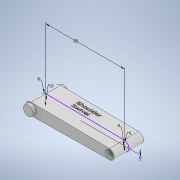
# Autodesk Inventor part: shoulder swivel
Saved by Autodesk Inventor 2020 (Build 240168000, 168)
## iProperties
Created: 2020-12-23
Part Number: shoulder swivel
Material: Generic
Document SubType Name: Modeling
Designer: frost
Density: 1 g/cm^3
Appearance: Default
Author: frost
Autodesk Inventor part; units mm, degrees
ref_plane "YZ Plane" through (0, 0, 0) normal (1, 0, 0) x (0, 1, 0)
ref_plane "XZ Plane" through (0, 0, 0) normal (0, 1, 0) x (-1, 0, 0)
ref_plane "XY Plane" through (0, 0, 0) normal (0, 0, 1) x (1, 0, 0)
sketch "Sketch1" plane through (0, 0, 0) normal (0, 0, 1) x (1, 0, 0)
  line L0 (0, 0) -> (-34.9606, 0)
  circle A0 centre (-34.9606, 0) radius 5
  circle A1 centre (45.0394, 0) radius 4
  arc A2 (-34.8856, 5.9995) -> (-34.8856, -5.9995) centre (-34.9606, 0) ccw
  arc A3 (45.1019, -4.9996) -> (45.1019, 4.9996) centre (45.0394, 0) ccw
  line L1 (-34.8856, 5.9995) -> (45.1019, 4.9996)
  line L2 (-34.8856, -5.9995) -> (45.1019, -4.9996)
  line L3 (-34.9606, 0) -> (-29.9606, 0)
  line L4 (-34.9606, 0) -> (-12.8373, 0)
  dimension "d7" = 10
  dimension "d6" = 6
  dimension "d8" = 8
  dimension "d9" = 5
  dimension "d10" = 80
  dimension "d15" = 0
  constraints: 10 end point, 4 point on circle, 4 tangent, 3 centre point, 3 coincident, 2 horizontal, 1 horizontal alignment, 1 point on line, 2 other
  measures "d6" radius of A2
  measures "d8" diameter of A1
  measures "d9" radius of A3
  measures "d10" distance of point (-34.961, 0) A1.centre
  measures "d15" distance from line of A1.centre L0
extrude "Extrusion1" add sketch "Sketch1" along normal mid plane 30
extrude "Extrusion2" add sketch "Sketch1" along normal mid plane 36 contours A0
sketch "Sketch2" plane through (-34.8856, 5.9995, 15) normal (0.0125, 0.9999219, 0) x (0.9999219, -0.0125, 0)
  line L0 (23.1356, 25.456) -> (63.8694, 25.456) construction
  line L1 (63.8694, 25.456) -> (63.8694, 9.0854) construction
  line L2 (63.8694, 9.0854) -> (23.1356, 9.0854) construction
  line L3 (23.1356, 9.0854) -> (23.1356, 25.456) construction
  spline S0 degree 2 poles (24.8731, 22.2157) (24.3763, 22.2157) (23.6769, 22.3541) (23.3704, 22.453) knots 0 0 0 1 2 2 2
  line L4 (23.3704, 22.453) -> (23.3704, 22.9621)
  line L5 (23.3704, 22.9621) -> (23.4124, 22.9621)
  spline S1 degree 2 poles (23.4124, 22.9621) (23.7139, 22.7743) (24.4777, 22.5667) (24.8311, 22.5667) knots 0 0 0 1 2 2 2
  spline S2 degree 2 poles (24.8311, 22.5667) (25.3353, 22.5667) (25.8519, 22.846) (25.8519, 23.0758) knots 0 0 0 1 2 2 2
  spline S3 degree 2 poles (25.8519, 23.0758) (25.8519, 23.2587) (25.5825, 23.4861) (25.2859, 23.543) knots 0 0 0 1 2 2 2
  spline S4 degree 2 poles (25.2859, 23.543) (25.0733, 23.5825) (24.7224, 23.6369) (24.4604, 23.6814) knots 0 0 0 1 2 2 2
  spline S5 degree 2 poles (24.4604, 23.6814) (24.2231, 23.7234) (23.8474, 23.8495) (23.7041, 23.9508) knots 0 0 0 1 2 2 2
  spline S6 degree 2 poles (23.7041, 23.9508) (23.5607, 24.0521) (23.405, 24.324) (23.405, 24.502) knots 0 0 0 1 2 2 2
  spline S7 degree 2 poles (23.405, 24.502) (23.405, 24.8727) (24.2725, 25.3745) (24.9448, 25.3745) knots 0 0 0 1 2 2 2
  spline S8 degree 2 poles (24.9448, 25.3745) (25.3304, 25.3745) (26.015, 25.2731) (26.3067, 25.1767) knots 0 0 0 1 2 2 2
  line L6 (26.3067, 25.1767) -> (26.3067, 24.6923)
  line L7 (26.3067, 24.6923) -> (26.2597, 24.6923)
  spline S9 degree 2 poles (26.2597, 24.6923) (26.0422, 24.8258) (25.3601, 25.0235) (24.9844, 25.0235) knots 0 0 0 1 2 2 2
  spline S10 degree 2 poles (24.9844, 25.0235) (24.5592, 25.0235) (24.0377, 24.759) (24.0377, 24.544) knots 0 0 0 1 2 2 2
  spline S11 degree 2 poles (24.0377, 24.544) (24.0377, 24.3512) (24.3442, 24.1213) (24.6383, 24.0694) knots 0 0 0 1 2 2 2
  spline S12 degree 2 poles (24.6383, 24.0694) (24.8311, 24.0348) (25.3897, 23.9459) (25.5751, 23.9088) knots 0 0 0 1 2 2 2
  spline S13 degree 2 poles (25.5751, 23.9088) (26.0472, 23.8124) (26.4846, 23.4243) (26.4846, 23.1401) knots 0 0 0 1 2 2 2
  spline S14 degree 2 poles (26.4846, 23.1401) (26.4846, 22.9597) (26.2671, 22.6136) (26.0694, 22.4925) knots 0 0 0 1 2 2 2
  spline S15 degree 2 poles (26.0694, 22.4925) (25.8494, 22.3591) (25.2908, 22.2157) (24.8731, 22.2157) knots 0 0 0 1 2 2 2
  line L8 (29.7571, 22.2701) -> (29.1787, 22.2701)
  line L9 (29.1787, 22.2701) -> (29.1787, 23.5751)
  spline S16 degree 2 poles (29.1787, 23.5751) (29.1787, 23.7333) (29.1318, 24.0052) (29.0675, 24.0867) knots 0 0 0 1 2 2 2
  spline S17 degree 2 poles (29.0675, 24.0867) (28.9983, 24.1732) (28.7462, 24.2573) (28.5262, 24.2573) knots 0 0 0 1 2 2 2
  spline S18 degree 2 poles (28.5262, 24.2573) (28.3112, 24.2573) (27.8539, 24.104) (27.6364, 23.9805) knots 0 0 0 1 2 2 2
  line L10 (27.6364, 23.9805) -> (27.6364, 22.2701)
  line L11 (27.6364, 22.2701) -> (27.0581, 22.2701)
  line L12 (27.0581, 22.2701) -> (27.0581, 25.456)
  line L13 (27.0581, 25.456) -> (27.6364, 25.456)
  line L14 (27.6364, 25.456) -> (27.6364, 24.3042)
  spline S19 degree 2 poles (27.6364, 24.3042) (27.8935, 24.46) (28.3977, 24.6231) (28.6795, 24.6231) knots 0 0 0 1 2 2 2
  spline S20 degree 2 poles (28.6795, 24.6231) (29.1861, 24.6231) (29.7571, 24.1782) (29.7571, 23.7555) knots 0 0 0 1 2 2 2
  line L15 (29.7571, 23.7555) -> (29.7571, 22.2701)
  spline S21 degree 2 poles (33.3904, 23.4144) (33.3904, 22.8361) (32.555, 22.2058) (31.8605, 22.2058) knots 0 0 0 1 2 2 2
  spline S22 degree 2 poles (31.8605, 22.2058) (31.1462, 22.2058) (30.3256, 22.8559) (30.3256, 23.4144) knots 0 0 0 1 2 2 2
  spline S23 degree 2 poles (30.3256, 23.4144) (30.3256, 23.9879) (31.1709, 24.6231) (31.8605, 24.6231) knots 0 0 0 1 2 2 2
  spline S24 degree 2 poles (31.8605, 24.6231) (32.555, 24.6231) (33.3904, 23.9903) (33.3904, 23.4144) knots 0 0 0 1 2 2 2
  spline S25 degree 2 poles (32.7947, 23.4144) (32.7947, 23.8593) (32.3103, 24.2919) (31.8605, 24.2919) knots 0 0 0 1 2 2 2
  spline S26 degree 2 poles (31.8605, 24.2919) (31.4106, 24.2919) (30.9212, 23.8593) (30.9212, 23.4144) knots 0 0 0 1 2 2 2
  spline S27 degree 2 poles (30.9212, 23.4144) (30.9212, 22.9819) (31.4106, 22.537) (31.8605, 22.537) knots 0 0 0 1 2 2 2
  spline S28 degree 2 poles (31.8605, 22.537) (32.3054, 22.537) (32.7947, 22.9745) (32.7947, 23.4144) knots 0 0 0 1 2 2 2
  line L16 (36.6579, 22.2701) -> (36.0795, 22.2701)
  line L17 (36.0795, 22.2701) -> (36.0795, 22.5222)
  spline S29 degree 2 poles (36.0795, 22.5222) (35.8126, 22.3665) (35.3331, 22.2058) (35.0365, 22.2058) knots 0 0 0 1 2 2 2
  spline S30 degree 2 poles (35.0365, 22.2058) (34.8141, 22.2058) (34.4161, 22.3047) (34.2703, 22.411) knots 0 0 0 1 2 2 2
  spline S31 degree 2 poles (34.2703, 22.411) (34.122, 22.5172) (33.9589, 22.841) (33.9589, 23.0734) knots 0 0 0 1 2 2 2
  line L18 (33.9589, 23.0734) -> (33.9589, 24.5588)
  line L19 (33.9589, 24.5588) -> (34.5372, 24.5588)
  line L20 (34.5372, 24.5588) -> (34.5372, 23.2538)
  spline S32 degree 2 poles (34.5372, 23.2538) (34.5372, 23.0709) (34.5768, 22.8311) (34.6485, 22.7422) knots 0 0 0 1 2 2 2
  spline S33 degree 2 poles (34.6485, 22.7422) (34.7177, 22.6532) (34.9624, 22.5716) (35.1898, 22.5716) knots 0 0 0 1 2 2 2
  spline S34 degree 2 poles (35.1898, 22.5716) (35.3998, 22.5716) (35.8793, 22.7323) (36.0795, 22.8484) knots 0 0 0 1 2 2 2
  line L21 (36.0795, 22.8484) -> (36.0795, 24.5588)
  line L22 (36.0795, 24.5588) -> (36.6579, 24.5588)
  line L23 (36.6579, 24.5588) -> (36.6579, 22.2701)
  line L24 (38.084, 22.2701) -> (37.5057, 22.2701)
  line L25 (37.5057, 22.2701) -> (37.5057, 25.456)
  line L26 (37.5057, 25.456) -> (38.084, 25.456)
  line L27 (38.084, 25.456) -> (38.084, 22.2701)
  line L28 (41.574, 22.2701) -> (40.9956, 22.2701)
  line L29 (40.9956, 22.2701) -> (40.9956, 22.5024)
  spline S35 degree 2 poles (40.9956, 22.5024) (40.8597, 22.4283) (40.6644, 22.3294) (40.531, 22.2874) knots 0 0 0 1 2 2 2
  spline S36 degree 2 poles (40.531, 22.2874) (40.4098, 22.2478) (40.1454, 22.2058) (39.9699, 22.2058) knots 0 0 0 1 2 2 2
  spline S37 degree 2 poles (39.9699, 22.2058) (39.6906, 22.2058) (39.2136, 22.3615) (39.048, 22.5123) knots 0 0 0 1 2 2 2
  spline S38 degree 2 poles (39.048, 22.5123) (38.8799, 22.6631) (38.6945, 23.108) (38.6945, 23.3971) knots 0 0 0 1 2 2 2
  spline S39 degree 2 poles (38.6945, 23.3971) (38.6945, 23.6987) (38.9269, 24.1386) (39.1345, 24.3042) knots 0 0 0 1 2 2 2
  spline S40 degree 2 poles (39.1345, 24.3042) (39.3223, 24.4525) (39.8537, 24.6231) (40.1454, 24.6231) knots 0 0 0 1 2 2 2
  spline S41 degree 2 poles (40.1454, 24.6231) (40.4024, 24.6231) (40.7831, 24.5465) (40.9956, 24.4674) knots 0 0 0 1 2 2 2
  line L30 (40.9956, 24.4674) -> (40.9956, 25.456)
  line L31 (40.9956, 25.456) -> (41.574, 25.456)
  line L32 (41.574, 25.456) -> (41.574, 22.2701)
  line L33 (40.9956, 22.8262) -> (40.9956, 24.1485)
  spline S42 degree 2 poles (40.9956, 24.1485) (40.7806, 24.2177) (40.4395, 24.2696) (40.2393, 24.2696) knots 0 0 0 1 2 2 2
  spline S43 degree 2 poles (40.2393, 24.2696) (39.7944, 24.2696) (39.2902, 23.8247) (39.2902, 23.4046) knots 0 0 0 1 2 2 2
  spline S44 degree 2 poles (39.2902, 23.4046) (39.2902, 22.9992) (39.6782, 22.5716) (40.1034, 22.5716) knots 0 0 0 1 2 2 2
  spline S45 degree 2 poles (40.1034, 22.5716) (40.3308, 22.5716) (40.793, 22.71) (40.9956, 22.8262) knots 0 0 0 1 2 2 2
  spline S46 degree 2 poles (43.8998, 22.2182) (43.0792, 22.2182) (42.1721, 22.8336) (42.1721, 23.4021) knots 0 0 0 1 2 2 2
  spline S47 degree 2 poles (42.1721, 23.4021) (42.1721, 23.9607) (43.052, 24.6231) (43.7614, 24.6231) knots 0 0 0 1 2 2 2
  spline S48 degree 2 poles (43.7614, 24.6231) (44.0802, 24.6231) (44.5721, 24.4995) (44.7575, 24.3685) knots 0 0 0 1 2 2 2
  spline S49 degree 2 poles (44.7575, 24.3685) (44.9404, 24.2375) (45.1381, 23.8593) (45.1381, 23.585) knots 0 0 0 1 2 2 2
  line L34 (45.1381, 23.585) -> (45.1381, 23.3749)
  line L35 (45.1381, 23.3749) -> (42.7579, 23.3749)
  spline S50 degree 2 poles (42.7579, 23.3749) (42.7579, 22.977) (43.361, 22.5543) (43.8924, 22.5543) knots 0 0 0 1 2 2 2
  spline S51 degree 2 poles (43.8924, 22.5543) (44.0827, 22.5543) (44.4485, 22.6112) (44.5968, 22.6557) knots 0 0 0 1 2 2 2
  spline S52 degree 2 poles (44.5968, 22.6557) (44.755, 22.7051) (44.97, 22.7916) (45.0392, 22.8311) knots 0 0 0 1 2 2 2
  line L36 (45.0392, 22.8311) -> (45.0738, 22.8311)
  line L37 (45.0738, 22.8311) -> (45.0738, 22.411)
  spline S53 degree 2 poles (45.0738, 22.411) (44.9725, 22.3838) (44.671, 22.3047) (44.5523, 22.2824) knots 0 0 0 1 2 2 2
  spline S54 degree 2 poles (44.5523, 22.2824) (44.3818, 22.2503) (44.1099, 22.2182) (43.8998, 22.2182) knots 0 0 0 1 2 2 2
  spline S55 degree 2 poles (44.5746, 23.669) (44.5696, 23.8247) (44.4707, 24.0521) (44.3768, 24.1288) knots 0 0 0 1 2 2 2
  spline S56 degree 2 poles (44.3768, 24.1288) (44.2755, 24.2153) (43.9591, 24.3067) (43.7268, 24.3067) knots 0 0 0 1 2 2 2
  spline S57 degree 2 poles (43.7268, 24.3067) (43.4945, 24.3067) (43.1731, 24.2153) (43.0397, 24.1263) knots 0 0 0 1 2 2 2
  spline S58 degree 2 poles (43.0397, 24.1263) (42.9111, 24.0348) (42.7752, 23.8149) (42.7579, 23.669) knots 0 0 0 1 2 2 2
  line L38 (42.7579, 23.669) -> (44.5746, 23.669)
  line L39 (47.5405, 24.1461) -> (47.5109, 24.1461)
  spline S59 degree 2 poles (47.5109, 24.1461) (47.4441, 24.1584) (47.3008, 24.1634) (47.1994, 24.1634) knots 0 0 0 1 2 2 2
  spline S60 degree 2 poles (47.1994, 24.1634) (46.9671, 24.1634) (46.5049, 24.0274) (46.2998, 23.8939) knots 0 0 0 1 2 2 2
  line L40 (46.2998, 23.8939) -> (46.2998, 22.2701)
  line L41 (46.2998, 22.2701) -> (45.7214, 22.2701)
  line L42 (45.7214, 22.2701) -> (45.7214, 24.5588)
  line L43 (45.7214, 24.5588) -> (46.2998, 24.5588)
  line L44 (46.2998, 24.5588) -> (46.2998, 24.2177)
  spline S61 degree 2 poles (46.2998, 24.2177) (46.6161, 24.4056) (47.0857, 24.5588) (47.3082, 24.5588) knots 0 0 0 1 2 2 2
  spline S62 degree 2 poles (47.3082, 24.5588) (47.3972, 24.5588) (47.4861, 24.5539) (47.5405, 24.5465) knots 0 0 0 1 2 2 2
  line L45 (47.5405, 24.5465) -> (47.5405, 24.1461)
  spline S63 degree 2 poles (24.8731, 17.194) (24.3763, 17.194) (23.6769, 17.3324) (23.3704, 17.4312) knots 0 0 0 1 2 2 2
  line L46 (23.3704, 17.4312) -> (23.3704, 17.9404)
  line L47 (23.3704, 17.9404) -> (23.4124, 17.9404)
  spline S64 degree 2 poles (23.4124, 17.9404) (23.7139, 17.7526) (24.4777, 17.5449) (24.8311, 17.5449) knots 0 0 0 1 2 2 2
  spline S65 degree 2 poles (24.8311, 17.5449) (25.3353, 17.5449) (25.8519, 17.8242) (25.8519, 18.0541) knots 0 0 0 1 2 2 2
  spline S66 degree 2 poles (25.8519, 18.0541) (25.8519, 18.237) (25.5825, 18.4644) (25.2859, 18.5212) knots 0 0 0 1 2 2 2
  spline S67 degree 2 poles (25.2859, 18.5212) (25.0733, 18.5608) (24.7224, 18.6152) (24.4604, 18.6596) knots 0 0 0 1 2 2 2
  spline S68 degree 2 poles (24.4604, 18.6596) (24.2231, 18.7017) (23.8474, 18.8277) (23.7041, 18.9291) knots 0 0 0 1 2 2 2
  spline S69 degree 2 poles (23.7041, 18.9291) (23.5607, 19.0304) (23.405, 19.3023) (23.405, 19.4802) knots 0 0 0 1 2 2 2
  spline S70 degree 2 poles (23.405, 19.4802) (23.405, 19.851) (24.2725, 20.3527) (24.9448, 20.3527) knots 0 0 0 1 2 2 2
  spline S71 degree 2 poles (24.9448, 20.3527) (25.3304, 20.3527) (26.015, 20.2514) (26.3067, 20.155) knots 0 0 0 1 2 2 2
  line L48 (26.3067, 20.155) -> (26.3067, 19.6705)
  line L49 (26.3067, 19.6705) -> (26.2597, 19.6705)
  spline S72 degree 2 poles (26.2597, 19.6705) (26.0422, 19.804) (25.3601, 20.0017) (24.9844, 20.0017) knots 0 0 0 1 2 2 2
  spline S73 degree 2 poles (24.9844, 20.0017) (24.5592, 20.0017) (24.0377, 19.7373) (24.0377, 19.5222) knots 0 0 0 1 2 2 2
  spline S74 degree 2 poles (24.0377, 19.5222) (24.0377, 19.3295) (24.3442, 19.0996) (24.6383, 19.0477) knots 0 0 0 1 2 2 2
  spline S75 degree 2 poles (24.6383, 19.0477) (24.8311, 19.0131) (25.3897, 18.9241) (25.5751, 18.887) knots 0 0 0 1 2 2 2
  spline S76 degree 2 poles (25.5751, 18.887) (26.0472, 18.7906) (26.4846, 18.4026) (26.4846, 18.1184) knots 0 0 0 1 2 2 2
  spline S77 degree 2 poles (26.4846, 18.1184) (26.4846, 17.9379) (26.2671, 17.5919) (26.0694, 17.4708) knots 0 0 0 1 2 2 2
  spline S78 degree 2 poles (26.0694, 17.4708) (25.8494, 17.3373) (25.2908, 17.194) (24.8731, 17.194) knots 0 0 0 1 2 2 2
  line L50 (31.2203, 19.5371) -> (30.3503, 17.2483)
  line L51 (30.3503, 17.2483) -> (29.8164, 17.2483)
  line L52 (29.8164, 17.2483) -> (28.9761, 19.0131)
  line L53 (28.9761, 19.0131) -> (28.1431, 17.2483)
  line L54 (28.1431, 17.2483) -> (27.6117, 17.2483)
  line L55 (27.6117, 17.2483) -> (26.7318, 19.5371)
  line L56 (26.7318, 19.5371) -> (27.3324, 19.5371)
  line L57 (27.3324, 19.5371) -> (27.9404, 17.7649)
  line L58 (27.9404, 17.7649) -> (28.7536, 19.5371)
  line L59 (28.7536, 19.5371) -> (29.2306, 19.5371)
  line L60 (29.2306, 19.5371) -> (30.0685, 17.7649)
  line L61 (30.0685, 17.7649) -> (30.6395, 19.5371)
  line L62 (30.6395, 19.5371) -> (31.2203, 19.5371)
  line L63 (32.3177, 17.2483) -> (31.7393, 17.2483)
  line L64 (31.7393, 17.2483) -> (31.7393, 19.5371)
  line L65 (31.7393, 19.5371) -> (32.3177, 19.5371)
  line L66 (32.3177, 19.5371) -> (32.3177, 17.2483)
  line L67 (32.3597, 19.9177) -> (31.7023, 19.9177)
  line L68 (31.7023, 19.9177) -> (31.7023, 20.3181)
  line L69 (31.7023, 20.3181) -> (32.3597, 20.3181)
  line L70 (32.3597, 20.3181) -> (32.3597, 19.9177)
  line L71 (35.8645, 19.5371) -> (34.5694, 17.2483)
  line L72 (34.5694, 17.2483) -> (34.0503, 17.2483)
  line L73 (34.0503, 17.2483) -> (32.7651, 19.5371)
  line L74 (32.7651, 19.5371) -> (33.3879, 19.5371)
  line L75 (33.3879, 19.5371) -> (34.3296, 17.7699)
  line L76 (34.3296, 17.7699) -> (35.2614, 19.5371)
  line L77 (35.2614, 19.5371) -> (35.8645, 19.5371)
  spline S79 degree 2 poles (37.7899, 17.1964) (36.9693, 17.1964) (36.0622, 17.8119) (36.0622, 18.3803) knots 0 0 0 1 2 2 2
  spline S80 degree 2 poles (36.0622, 18.3803) (36.0622, 18.9389) (36.9421, 19.6013) (37.6515, 19.6013) knots 0 0 0 1 2 2 2
  spline S81 degree 2 poles (37.6515, 19.6013) (37.9703, 19.6013) (38.4622, 19.4778) (38.6476, 19.3468) knots 0 0 0 1 2 2 2
  spline S82 degree 2 poles (38.6476, 19.3468) (38.8305, 19.2158) (39.0282, 18.8376) (39.0282, 18.5632) knots 0 0 0 1 2 2 2
  line L78 (39.0282, 18.5632) -> (39.0282, 18.3532)
  line L79 (39.0282, 18.3532) -> (36.648, 18.3532)
  spline S83 degree 2 poles (36.648, 18.3532) (36.648, 17.9552) (37.2511, 17.5326) (37.7825, 17.5326) knots 0 0 0 1 2 2 2
  spline S84 degree 2 poles (37.7825, 17.5326) (37.9728, 17.5326) (38.3386, 17.5894) (38.4869, 17.6339) knots 0 0 0 1 2 2 2
  spline S85 degree 2 poles (38.4869, 17.6339) (38.6451, 17.6833) (38.8601, 17.7699) (38.9293, 17.8094) knots 0 0 0 1 2 2 2
  line L80 (38.9293, 17.8094) -> (38.9639, 17.8094)
  line L81 (38.9639, 17.8094) -> (38.9639, 17.3892)
  spline S86 degree 2 poles (38.9639, 17.3892) (38.8626, 17.362) (38.5611, 17.2829) (38.4424, 17.2607) knots 0 0 0 1 2 2 2
  spline S87 degree 2 poles (38.4424, 17.2607) (38.2719, 17.2286) (38, 17.1964) (37.7899, 17.1964) knots 0 0 0 1 2 2 2
  spline S88 degree 2 poles (38.4647, 18.6473) (38.4597, 18.803) (38.3609, 19.0304) (38.2669, 19.107) knots 0 0 0 1 2 2 2
  spline S89 degree 2 poles (38.2669, 19.107) (38.1656, 19.1935) (37.8492, 19.285) (37.6169, 19.285) knots 0 0 0 1 2 2 2
  spline S90 degree 2 poles (37.6169, 19.285) (37.3846, 19.285) (37.0633, 19.1935) (36.9298, 19.1045) knots 0 0 0 1 2 2 2
  spline S91 degree 2 poles (36.9298, 19.1045) (36.8013, 19.0131) (36.6653, 18.7931) (36.648, 18.6473) knots 0 0 0 1 2 2 2
  line L82 (36.648, 18.6473) -> (38.4647, 18.6473)
  line L83 (40.2022, 17.2483) -> (39.6239, 17.2483)
  line L84 (39.6239, 17.2483) -> (39.6239, 20.4343)
  line L85 (39.6239, 20.4343) -> (40.2022, 20.4343)
  line L86 (40.2022, 20.4343) -> (40.2022, 17.2483)
  point P0 (34.9579, 15)
  constraints: 2 other
extrude "Extrusion3" cut sketch "Sketch2" against normal blind 5
body "Solid1"
